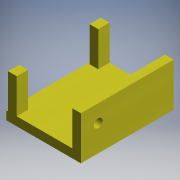
# Autodesk Inventor part: Upper_leg
Saved by Autodesk Inventor 2017 (Build 210142000, 142)
## iProperties
Part Number: Upper_leg
Material: Generic
Document SubType Name: Modeling
Designer: alex-
Appearance: Canary
Author: alex-
Autodesk Inventor part; units mm, degrees
ref_plane "YZ Plane" through (0, 0, 0) normal (1, 0, 0) x (0, 1, 0)
ref_plane "XZ Plane" through (0, 0, 0) normal (0, 1, 0) x (-1, 0, 0)
ref_plane "XY Plane" through (0, 0, 0) normal (0, 0, 1) x (1, 0, 0)
sketch "Sketch8" plane through (0, 0, 0) normal (0, 1, 0) x (-1, 0, 0)
  line L0 (21.5, 26.75) -> (-21.5, 26.75)
  line L1 (-21.5, 26.75) -> (-21.5, -26.75)
  line L2 (-21.5, -26.75) -> (21.5, -26.75)
  line L3 (21.5, -26.75) -> (21.5, 26.75)
  point P0 (0, 0)
  point P1 (0, 26.75)
  point P2 (21.5, 0)
  dimension "d31" = 43
  dimension "d32" = 53.5
  constraints: 8 end point, 2 midpoint, 2 parallel, 1 horizontal, 1 horizontal alignment, 1 perpendicular, 1 vertical alignment
  measures "d31" distance of L0.start L0.end
  measures "d32" distance of L2.end L0.start
extrude "Extrusion8" add sketch "Sketch8" along normal blind 5
sketch "Sketch9" plane through (0, 5, 0) normal (0, 1, 0) x (1, 0, 0)
  line L0 (-20.5, -26.75) -> (-15.5, -26.75)
  line L1 (-15.5, -26.75) -> (-15.5, -20.25)
  line L2 (-15.5, -20.25) -> (-20.5, -20.25)
  line L3 (-20.5, -20.25) -> (-20.5, -26.75)
  line L4 (-20.5, 20.25) -> (-15.5, 20.25)
  line L5 (-15.5, 20.25) -> (-15.5, 26.75)
  line L6 (-15.5, 26.75) -> (-20.5, 26.75)
  line L7 (-20.5, 26.75) -> (-20.5, 20.25)
  line L8 (-21.5, -26.75) -> (21.5, -26.75) projected
  line L9 (21.5, 26.75) -> (-21.5, 26.75) projected
  line L10 (-21.5, 26.75) -> (-21.5, -26.75) projected
  line L11 (16.5, -26.75) -> (21.5, -26.75)
  line L12 (21.5, -26.75) -> (21.5, 26.75)
  line L13 (21.5, 26.75) -> (16.5, 26.75)
  line L14 (16.5, 26.75) -> (16.5, -26.75)
  line L15 (21.5, -26.75) -> (21.5, 26.75) projected
  point P0 (0, 0)
  point P1 (-18, -26.75)
  point P2 (-18, 26.75)
  point P3 (19, -26.75)
  point P4 (19, 26.75)
  point P5 (21.5, 0)
  dimension "d35" = 6.5
  dimension "d36" = 5
  dimension "d38" = 6
  dimension "d41" = 5
  constraints: 24 end point, 6 midpoint, 6 parallel, 4 point on line, 3 horizontal, 3 perpendicular, 2 equal length, 1 vertical alignment
  measures "d35" distance of L2.end L0.start
  measures "d36" distance of L1.end L2.end
  measures "d38" distance between parallel lines of L1 L10
  measures "d41" distance between parallel lines of L14 L12
extrude "Extrusion9" add sketch "Sketch9" along normal blind 20 contours L3 L2 L1 L0 | L14 L9 L12 L8 | L6 L5 L4 L7
sketch "Sketch10" plane through (21.5, 0, 26.75) normal (1, 0, 0) x (0, 0, -1)
  circle A0 centre (10, 15) radius 2.5
  line L0 (0, 25) -> (53.5, 25) projected
  line L1 (0, 0) -> (0, 25) projected
  point P0 (26.75, 0)
  dimension "d42" = 5
  dimension "d43" = 10
  dimension "d44" = 10
  constraints: 1 centre point
  measures "d42" diameter of A0
  measures "d43" distance from line of A0.centre L0
  measures "d44" distance from line of A0.centre L1
extrude "Extrusion10" cut sketch "Sketch10" against normal up to next
equation "\"d31\" = s_height + b_mat_thickness"
equation "\"d32\" = s_width + 2 * s_land"
equation "\"d33\" = b_mat_thickness"
equation "\"d35\" = s_land"
equation "\"d36\" = b_mat_thickness"
equation "\"d38\" = s_land_dist_top - s_land_pin_thickness"
equation "\"d41\" = b_mat_thickness"
equation "\"d39\" = s_depth"
equation "\"d43\" = 0.5 * s_depth"
equation "\"d44\" = s_shaft_front_dist"
equation "\"s_height\" = 38"
equation "\"b_mat_thickness\" = 5"
equation "\"s_width\" = 40.5"
equation "\"s_land\" = 6.5"
equation "\"s_land_dist_top\" = 8"
equation "\"s_land_pin_thickness\" = 2"
equation "\"s_depth\" = 20"
equation "\"s_shaft_front_dist\" = 10"
body "Solid2"
